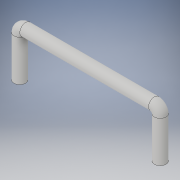
# Autodesk Inventor part: bus bar
Saved by Autodesk Inventor 2019.3 (Build 233278000, 278)
## iProperties
Created: 2019-11-25
Part Number: bus bar
Material: Generic
Document SubType Name: Modeling
Designer: kjdix
Density: 1 g/cm^3
Appearance: Default
Author: kjdix
Autodesk Inventor part; units mm, degrees
ref_plane "YZ Plane" through (0, 0, 0) normal (1, 0, 0) x (0, 1, 0)
ref_plane "XZ Plane" through (0, 0, 0) normal (0, 1, 0) x (-1, 0, 0)
ref_plane "XY Plane" through (0, 0, 0) normal (0, 0, 1) x (1, 0, 0)
sketch "Sketch1" plane through (0, 0, 0) normal (0, 1, 0) x (-1, 0, 0)
  line L0 (0, 0) -> (-7.62, 0) construction
  line L1 (0, 0) -> (7.62, 0) construction
  circle A0 centre (7.62, 0) radius 0.635
  dimension "d0" = 7.62
  dimension "d1" = 7.62
  dimension "d2" = 1.27
  constraints: 4 end point, 2 horizontal, 1 centre point, 1 coincident
  measures "d0" distance of L0.start L0.end
  measures "d1" distance of L0.start L1.end
  measures "d2" diameter of A0
sketch "Sketch2" plane through (0, 0, 0) normal (0, 0, 1) x (1, 0, 0)
  line L0 (0, 0) -> (-7.62, 0) construction
  line L1 (0, 0) -> (7.62, 0) construction
  line L2 (-7.62, 0) -> (-7.62, 1.905)
  arc A0 (-6.985, 2.54) -> (-7.62, 1.905) centre (-6.985, 1.905) ccw
  line L3 (7.62, 0) -> (7.62, 1.905)
  line L4 (6.985, 2.54) -> (-6.985, 2.54)
  arc A1 (7.62, 1.905) -> (6.985, 2.54) centre (6.985, 1.905) ccw
  point P0 (-7.62, 2.54)
  point P1 (3.81, 2.54)
  point P2 (7.62, 2.54)
  dimension "d3" = 2.54
  dimension "d5" = 0.635
  dimension "d10" = 2.54
  dimension "d11" = 0.635
  constraints: 6 end point, 4 point on circle, 3 point on line, 3 tangent, 2 centre point, 2 vertical, 1 perpendicular
  measures "d3" distance of L0.end point (-7.62, 2.54)
  measures "d5" radius of A0
  measures "d10" distance of L1.end point (7.62, 2.54)
  measures "d11" radius of A1
sweep "Sweep1" add profiles "Sketch1" path "Sketch2" path curves L2 A0 L4 A1 L3
sketch "Sketch3" plane through (-7.62, 0, 0) normal (0, -1, 0) x (1, 0, 0)
  circle A0 centre (0, 0) radius 0.635 projected
  circle A1 centre (15.24, 0) radius 0.635 projected
  point P0 (7.62, 0)
extrude "Extrusion1" add sketch "Sketch3" along normal blind 2.54
body "Solid1"
